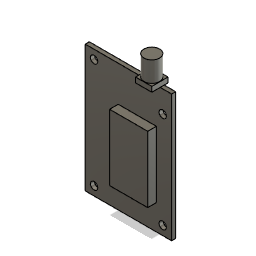
RN2483 v2 (Autodesk Fusion 360 design; units mm, degrees)
Autodesk Fusion 360 part; units mm, degrees
sketch "Sketch1" plane through (0, 0, 0) normal (0, 0, 1) x (1, 0, 0)
  line L0 (17, 25) -> (-17, 25)
  line L1 (-17, 25) -> (-17, -25)
  line L2 (-17, -25) -> (17, -25)
  line L3 (17, -25) -> (17, 25)
  line L4 (17, 25) -> (-17, -25) construction
  line L5 (-17, 25) -> (17, -25) construction
  circle A0 centre (-13.5, 21.5) radius 1.45
  line L6 (-20, 0) -> (19, 0) construction
  circle A1 centre (-13.5, -21.5) radius 1.45
  line L7 (0, -29) -> (0, 26) construction
  circle A2 centre (13.5, -21.5) radius 1.45
  circle A3 centre (13.5, 16.4) radius 1.45
  line L8 (-4, 11) -> (11, 11)
  line L9 (11, 11) -> (11, -15)
  line L10 (11, -15) -> (-4, -15)
  line L11 (-4, -15) -> (-4, 11)
  dimension "d1" = 34
  dimension "d2" = 50
  dimension "d3" = 2.9
  dimension "d4" = 3.5
  dimension "d5" = 3.5
  dimension "d6" = 2.9
  dimension "d7" = 3.5
  dimension "d8" = 8.6
  constraint horizontal L0
  constraint perpendicular L0 L1
  constraint parallel L0 L2
  constraint parallel L1 L3
  constraint coincident L4 origin
  constraint coincident L5 origin
  constraint perpendicular L3 L6
  constraint symmetric A0 L6 A1
  constraint perpendicular L0 L7
  constraint symmetric A1 L7 A2
  constraint horizontal L8
  constraint vertical L9
  constraint horizontal L10
  constraint vertical L11
  measures "d1" distance of L1.end L2.end
  measures "d2" distance of L0.end L1.end
  measures "d3" diameter of A0
  measures "d4" distance of L0 A0.centre
  measures "d5" distance of L1 A0.centre
  measures "d6" diameter of A3
  measures "d7" distance of L3 A3.centre
  measures "d8" distance of L0 A3.centre
extrude "Extrude1" add sketch "Sketch1" along normal blind 1.6 contours L0 L1 L2 L3 | L8 L9 L10 L11
extrude "Extrude2" add sketch "Sketch1" along normal blind 5 contours L8 L9 L10 L11
sketch "Sketch2" plane through (0, 25, 0) normal (0, 1, 0) x (-1, 0, 0)
  line L0 (-17, 0) -> (17, 0)
  line L1 (17, 0) -> (17, 1.6)
  line L2 (17, 1.6) -> (-17, 1.6)
  line L3 (-17, 1.6) -> (-17, 0)
  line L4 (-6.1, -1.5) -> (-12.5, -1.5)
  line L5 (-12.5, -1.5) -> (-12.5, 4.9)
  line L6 (-12.5, 4.9) -> (-6.1, 4.9)
  line L7 (-6.1, 4.9) -> (-6.1, -1.5)
  line L8 (-17, 0) -> (17, 0)
  line L9 (-6.1, -1.5) -> (-12.5, 4.9) construction
  line L10 (-12.5, -1.5) -> (-6.1, 4.9) construction
  circle A0 centre (-9.3, 1.7) radius 3.1
  dimension "d13" = 6.4
  dimension "d14" = 6.4
  dimension "d15" = 4.5
  dimension "d16" = 1.5
  dimension "d17" = 6.2
  constraint horizontal L4
  constraint vertical L5
  constraint horizontal L6
  constraint vertical L7
  constraint midpoint L9 A0.centre
  measures "d13" distance of L4.start L4.end
  measures "d14" distance of L4.start L6.end
  measures "d15" distance of L3 L5
  measures "d16" distance of L4 L8
  measures "d17" diameter of A0
extrude "Extrude3" add sketch "Sketch2" along normal blind 2 contours L0 L2 L5 L8 A0 | L0 L4 L5 L7 L8 A0 | L0 L2 L8 A0 | L0 L8 A0 | L2 L5 L6 L7 A0 | L0 L2 L7 L8 A0 | L2 A0
extrude "Extrude4" add sketch "Sketch2" along normal blind 10 contours L0 L2 L8 A0 | L0 L8 A0 | L2 A0
equation "d4 = 2 mm + 1.5 mm"
equation "d8 = 7.1 mm + 1.5 mm"
